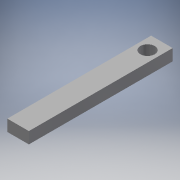
# Autodesk Inventor part: pendulum
Saved by Autodesk Inventor 2017 (Build 210142000, 142)
## iProperties
Created: 2022-03-10
Part Number: pendulum
Material: Stahl
Document SubType Name: Modeling
Designer: 10154704
Density: 7.85 g/cm^3
Appearance: Stahl
Author: 10154704
Autodesk Inventor part; units mm, degrees
ref_plane "YZ Plane" through (0, 0, 0) normal (1, 0, 0) x (0, 1, 0)
ref_plane "XZ Plane" through (0, 0, 0) normal (0, 1, 0) x (-1, 0, 0)
ref_plane "XY Plane" through (0, 0, 0) normal (0, 0, 1) x (1, 0, 0)
sketch "Skizze1" plane through (0, 0, 0) normal (0, 0, 1) x (1, 0, 0)
  line L0 (-7.5, 10) -> (7.5, 10)
  line L1 (7.5, 10) -> (7.5, -90)
  line L2 (7.5, -90) -> (-7.5, -90)
  line L3 (-7.5, -90) -> (-7.5, 10)
  circle A0 centre (0, 0) radius 5
  dimension "d0" = 15
  dimension "d1" = 10
  dimension "d2" = 7.5
  dimension "d3" = 100
  dimension "d4" = 10
  constraints: 8 end point, 2 parallel, 1 centre point, 1 coincident, 1 horizontal, 1 perpendicular
  measures "d0" distance between parallel lines of L1 L3
  measures "d1" distance from line of point (0, 0) L0
  measures "d2" distance from line of L1 point (0, 0)
  measures "d3" distance between parallel lines of L2 L0
  measures "d4" diameter of A0
extrude "Extrusion1" add sketch "Skizze1" along normal blind 8
equation "\"d2\" = 0.5 * d0"
